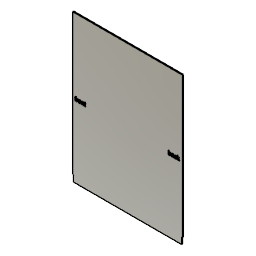
panel_3X8X (Autodesk Fusion 360 design; units mm, degrees)
part number: Configuration 1
Autodesk Fusion 360 part; units mm, degrees
sketch "MasterSketch" plane through (0, 0, 0) normal (0, 1, 0) x (1, 0, 0)
  line L0 (-711.2, -1930.4) -> (711.2, -1930.4)
  line L1 (711.2, -25.4) -> (-711.2, -25.4)
  line L2 (-711.2, -25.4) -> (-711.2, -1930.4)
  line L3 (0, -25.4) -> (0, 0) construction
  line L4 (711.2, -25.4) -> (711.2, -1930.4)
  line L5 (-711.2, -109.474) -> (-700.024, -109.474)
  line L6 (-700.024, -109.474) -> (-700.024, -25.4)
  line L7 (711.2, -109.474) -> (700.024, -109.474)
  line L8 (700.024, -109.474) -> (700.024, -25.4)
  dimension "d10" = 25.4
  dimension "d12" = 1422.4
  dimension "d259" = 1905
  dimension "d260" = 84.074
  dimension "d261" = 11.176
  dimension "d263" = 84.074
  dimension "d264" = 11.176
  constraint midpoint L1 L3.start
  constraint coincident L3.end origin
  constraint vertical L3
  constraint coincident L1 L4.start
  constraint coincident L0 L4.end
  constraint horizontal L0
  constraint coincident L1.start L4.start
  constraint coincident L0.end L4.end
  constraint coincident L2 L5.start
  constraint perpendicular L2 L5
  constraint coincident L1 L6.end
  constraint perpendicular L1 L6
  constraint coincident L4 L7.start
  constraint coincident L1 L8.end
  constraint perpendicular L1 L8
  constraint horizontal L1
  constraint perpendicular L0 L2
  constraint perpendicular L0 L4
  constraint perpendicular L7 L8
  measures "d10" distance of L3.start L3.end
  measures "d12" distance of L1.start L1.end
  measures "d259" distance of L0.start L1.end
  measures "d260" distance of L5.end L6.end
  measures "d261" distance of L5.start L5.end
  measures "d263" distance of L7.end L8.end
  measures "d264" distance of L7.start L7.end
extrude "panel_extrude" add sketch "MasterSketch" along normal mid plane 12.7 makes body 1 in component "3x8x_panel"
sketch "Labels_left" plane through (0, 0, 0) normal (0, 1, 0) x (1, 0, 0)
  line L0 (711.2, -25.4) -> (-711.2, -1930.4) construction
  line L1 (711.2, -1930.4) -> (-711.2, -25.4) construction
  line L2 (139.7, -901.7) -> (-139.7, -1054.1) construction
  line L3 (-139.7, -901.7) -> (139.7, -901.7) construction
  line L4 (139.7, -901.7) -> (139.7, -1054.1) construction
  line L5 (139.7, -1054.1) -> (-139.7, -1054.1) construction
  line L6 (-139.7, -1054.1) -> (-139.7, -901.7) construction
  line L7 (-708.025, -927.1) -> (-504.825, -927.1) construction
  line L8 (-504.825, -927.1) -> (-504.825, -1028.7) construction
  line L9 (-504.825, -1028.7) -> (-708.025, -1028.7) construction
  line L10 (-708.025, -1028.7) -> (-708.025, -927.1) construction
  line L11 (-711.2, -1930.4) -> (-711.2, -25.4) construction
  line L12 (-708.025, -977.9) -> (-711.2, -977.9)
  line L13 (0, 0) -> (0, -977.9) construction
  line L14 (504.825, -927.1) -> (708.025, -927.1) construction
  line L15 (708.025, -927.1) -> (708.025, -1028.7) construction
  line L16 (708.025, -1028.7) -> (504.825, -1028.7) construction
  line L17 (504.825, -1028.7) -> (504.825, -927.1) construction
  line L18 (711.2, -1930.4) -> (711.2, -25.4) construction
  line L19 (708.025, -977.9) -> (711.2, -977.9)
  point P0 (-711.2, -1930.4)
  point P1 (711.2, -1930.4)
  point P2 (711.2, -25.4)
  point P3 (-711.2, -25.4)
  point P4 (0, -977.9)
  dimension "d78" = 50.8
  dimension "d220" = 279.4
  dimension "d221" = 152.4
  dimension "d275" = 50.8
  dimension "d277" = 203.2
  dimension "d278" = 101.6
  dimension "d279" = 3.175
  dimension "d280" = 50.8
  dimension "d282" = 203.2
  dimension "d283" = 101.6
  dimension "d284" = 3.175
  text T0 "front" font "Arial" height 50.8 align centre middle in box 203.2 x 101.6 at (-708.025, -927.1) x (1, 0) y (0, -1) spacing 1 kerned
  text T1 "back" font "Arial" height 50.8 align centre middle in box 203.2 x 101.6 at (504.825, -927.1) x (1, 0) y (0, -1) spacing 1 kerned
  constraint coincident P2 L0.start
  constraint coincident P0 L0.end
  constraint coincident P1 L1.start
  constraint coincident P3 L1.end
  constraint coincident L0 P4
  constraint coincident L1 P4
  constraint midpoint P4 L2
  constraint horizontal L5
  constraint coincident L2.start
  constraint coincident L2.end
  constraint horizontal L9
  constraint midpoint L10 L12.start
  constraint midpoint L11 L12.end
  constraint perpendicular L11 L12
  constraint coincident L13.start origin
  constraint coincident P4 L13.end
  constraint horizontal L16
  constraint midpoint L15 L19.start
  constraint midpoint L18 L19.end
  constraint perpendicular L18 L19
  measures "d279" distance of L12.start L12.end
  measures "d284" distance of L15 L18
sketch "Labels_right" plane through (0, 0, 0) normal (0, 1, 0) x (1, 0, 0)
  line L0 (708.025, -977.9037) -> (711.2, -977.9)
  line L1 (707.9659, -927.1037) -> (504.766, -927.3403) construction
  line L2 (504.766, -927.3403) -> (504.8843, -1028.9403) construction
  line L3 (504.8843, -1028.9403) -> (708.0841, -1028.7037) construction
  line L4 (708.0841, -1028.7037) -> (707.9659, -927.1037) construction
  line L5 (-504.7389, -927.4509) -> (-707.9386, -927.1055) construction
  line L6 (-707.9386, -927.1055) -> (-708.1114, -1028.7053) construction
  line L7 (-708.1114, -1028.7053) -> (-504.9117, -1029.0507) construction
  line L8 (-504.9117, -1029.0507) -> (-504.7389, -927.4509) construction
  line L9 (-708.025, -977.9054) -> (-711.2, -977.9)
  line L10 (711.2, -1930.4) -> (711.2, -25.4) construction
  line L11 (-711.2, -1930.4) -> (-711.2, -25.4) construction
  point P0 (-711.2, -1930.4)
  point P1 (711.2, -1930.4)
  point P2 (711.2, -25.4)
  point P3 (-711.2, -25.4)
  dimension "d285" = 50.8
  dimension "d287" = 50.8
  dimension "d289" = 203.2
  dimension "d290" = 101.6
  dimension "d291" = 3.175
  dimension "d292" = 203.2
  dimension "d293" = 101.6
  dimension "d294" = 3.175
  text T0 "back" font "Arial" height 50.8 align centre middle in box 203.2 x 101.6 at (707.9659, -927.1037) x (-0.999999, -0.001164) y (0.001164, -0.999999) spacing 1 kerned
  text T1 "front" font "Arial" height 50.8 align centre middle in box 203.2 x 101.6 at (-504.7389, -927.4509) x (-0.999999, 0.0017) y (-0.0017, -0.999999) spacing 1 kerned
  constraint midpoint L0.start L4
  constraint midpoint L9.start L6
  constraint coincident P1 L10.start
  constraint coincident P2 L10.end
  constraint coincident P0 L11.start
  constraint coincident P3 L11.end
  constraint perpendicular L6 L9
  constraint midpoint L9.end L11
  constraint perpendicular L0 L4
  constraint midpoint L0.end L10
  measures "d291" distance of L0.start L0.end
  measures "d294" distance of L9.start L9.end
extrude "label_extrude" add sketch "Labels_left" against normal blind 3.175 from surface at -9.525 separate body text T0 T1 makes body 2 at (601.0985, -9.525, 962.947) makes body 3 at (-651.0916, -9.525, 971.189) makes body 4 at (615.939, -9.525, 959.7654) makes body 5 at (-667.1933, -9.525, 973.7995) makes body 6 at (-629.4646, -9.525, 973.4432) makes body 7 at (535.8638, -9.525, 976.2756) makes body 8 at (-545.2525, -9.525, 970.2188) makes body 9 at (650.5025, -9.525, 976.7103) makes body 10 at (-587.9208, -9.525, 971.4663) in component "LeftLabel"
extrude "Extrude1" add sketch "Labels_right" along normal blind 3.175 from surface at 9.525 separate body text T0 T1 makes body 11 at (-561.7472, 9.525, 971.4431) makes body 12 at (-583.3781, 9.525, 973.6604) makes body 13 at (676.9843, 9.525, 976.3154) makes body 14 at (562.3462, 9.525, 976.8836) makes body 15 at (596.89, 9.525, 959.8985) makes body 16 at (611.7342, 9.525, 963.0628) makes body 17 at (-624.9184, 9.525, 971.6129) makes body 18 at (-667.5845, 9.525, 970.2929) makes body 19 at (-543.5824, 9.525, 974.0844) in component "RightLabel"
extrude "left_notch" add sketch "MasterSketch" along normal mid plane 12.7 separate body contours L1 L2 L5 L6 makes body 20 in component "CutGeometry"
extrude "right_notch" add sketch "MasterSketch" along normal mid plane 12.7 separate body contours L1 L4 L7 L8 makes body 21 in component "CutGeometry"
combine "notch_boolean" operation cut target body 1 tool bodies 20 21 in component "3x8x_panel"
fillet "Fillet1" radius 6.35 2 edges at (700.024, 0, 109.474) (-700.024, 0, 109.474) on bodies 1 in component "3x8x_panel"
component "3x8x_panel" placed x (1, 0, 0) y (0, 1, 0) z (0, 0, 1) at (0, 0, 0)
component "LeftLabel" placed x (1, 0, 0) y (0, 1, 0) z (0, 0, 1) at (0, 0, 0)
component "RightLabel" placed x (1, 0, 0) y (0, 1, 0) z (0, 0, 1) at (0, 0, 0)
component "CutGeometry" placed x (1, 0, 0) y (0, 1, 0) z (0, 0, 1) at (0, 0, 0)
equation "component_height = 75 in" comment "001) Input - Model     Height of the component"
equation "component_width = 56 in" comment "002) Input - Model     Width of the component in inches"
equation "d10 = component_floor_clearance"
equation "d12 = component_width"
equation "component_thickness = 0.5 in" comment "006) Fixed - Model     Thickness of the component"
equation "d39 = component_thickness"
equation "d79 = 'left surface'"
equation "d82 = ( 1 / 8 ) * 1 in"
equation "d83 = ( 1 / 8 ) * 1 in"
equation "front_notching_activation_offset = if(notching_front_edge; 0 in; component_thickness)" comment "103) Derived - Helper     An offset that repositions a void relative to the panel, allowing the void to cut into the panel at the specified location and create the front notch in the model"
equation "back_notching_activation_offset = if(notching_back_edge; 0 in; component_thickness)" comment "104) Derived - Helper     An offset that repositions a void relative to the panel, allowing the void to cut into the panel at the specified location and create the back notch in the model"
equation "component_floor_clearance = 1 in" comment "003) Input - Model     Floor clearance of the component"
equation "notching_y_dist = 3.31 in" comment "008) Fixed - Model     Vertical height of notch"
equation "notching_front_edge = if(panel_inline_front and component_floor_clearance == 1 in; 1; 0)" comment "101) Derived - Model     Whether notching is present the front edge of the panel"
equation "notching_back_edge = if(panel_inline_back and component_floor_clearance == 1 in; 1; 0)" comment "102) Derived - Model     Whether notching is present the back edge of the panel"
equation "d259 = component_height"
equation "d260 = notching_y_dist"
equation "d261 = notching_x_dist"
equation "notching_x_dist = 0.44 in" comment "007) Fixed - Model     Horizontal length of notch"
equation "d263 = notching_y_dist"
equation "d264 = notching_x_dist"
equation "d265 = component_thickness"
equation "d267 = front_notching_activation_offset"
equation "d268 = back_notching_activation_offset"
equation "d269 = component_thickness"
equation "panel_inline_front = 1" comment "004) Input - Helper     Whether the panel's front edge attaches inline to a stile"
equation "panel_inline_back = 1" comment "005) Input - Helper     Whether the panel's back edge attaches inline to a stile"
equation "d276 = 'front'"
equation "d279 = ( 1 / 8 ) * 1 in"
equation "d281 = 'back'"
equation "d284 = d279"
equation "d286 = 'back'"
equation "d288 = 'front'"
equation "d291 = ( 1 / 8 ) * 1 in"
equation "d295 = ( 1 / 8 ) * 1 in"
equation "d296 = ( 1 / 8 ) * 1 in"
named bodies: "FrontNotch", "BackNotch"
